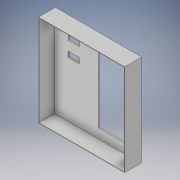
# Autodesk Inventor part: tetris body
Saved by Autodesk Inventor 2017 (Build 210142000, 142)
## iProperties
Created: 2019-08-23
Part Number: tetris body
Material: Generic
Document SubType Name: Modeling
Designer: EDMU0006
Density: 1 g/cm^3
Appearance: Default
Author: EDMU0006
Autodesk Inventor part; units mm, degrees
ref_plane "YZ Plane" through (0, 0, 0) normal (1, 0, 0) x (0, 1, 0)
ref_plane "XZ Plane" through (0, 0, 0) normal (0, 1, 0) x (-1, 0, 0)
ref_plane "XY Plane" through (0, 0, 0) normal (0, 0, 1) x (1, 0, 0)
sketch "Sketch1" plane through (0, 0, 0) normal (0, 0, 1) x (1, 0, 0)
  line L0 (-362.4815, -406.4) -> (399.5185, -406.4)
  line L1 (399.5185, -406.4) -> (399.5185, 406.4)
  line L2 (399.5185, 406.4) -> (-362.4815, 406.4)
  line L3 (-362.4815, 406.4) -> (-362.4815, -406.4)
  point P0 (0, 0)
  constraints: 8 end point, 2 perpendicular, 1 vertical
extrude "Extrusion1" add sketch "Sketch1" along normal blind 150.114
sketch "Sketch3" plane through (0, 0, 150.114) normal (0, 0, 1) x (1, 0, 0)
  line L0 (-356.7823, 401.8579) -> (395.0577, 401.8579)
  line L1 (395.0577, 401.8579) -> (395.0577, -400.7821)
  line L2 (395.0577, -400.7821) -> (-356.7823, -400.7821)
  line L3 (-356.7823, -400.7821) -> (-356.7823, 401.8579)
  point P0 (0, 0)
  dimension "d10" = 751.84
  dimension "d11" = 802.64
  constraints: 8 end point, 2 parallel, 1 horizontal, 1 perpendicular
  measures "d10" distance of L0.start L0.end
  measures "d11" distance of L0.end L1.end
extrude "Extrusion2" cut sketch "Sketch3" against normal blind 139.7
sketch "Sketch4" plane through (0, 0, 0) normal (0, 0, -1) x (-1, 0, 0)
  line L0 (-345.9489, 321.1782) -> (-25.9089, 321.1782)
  line L1 (-25.9089, 321.1782) -> (-25.9089, -318.9018)
  line L2 (-25.9089, -318.9018) -> (-345.9489, -318.9018)
  line L3 (-345.9489, -318.9018) -> (-345.9489, 321.1782)
  line L4 (140.3393, 137.685) -> (240.6693, 137.685)
  line L5 (240.6693, 137.685) -> (240.6693, 90.4401)
  line L6 (240.6693, 90.4401) -> (140.3393, 90.4401)
  line L7 (140.3393, 90.4401) -> (140.3393, 137.685)
  line L8 (139.7596, 266.0514) -> (240.0896, 266.0514)
  line L9 (240.0896, 266.0514) -> (240.0896, 218.8065)
  line L10 (240.0896, 218.8065) -> (139.7596, 218.8065)
  line L11 (139.7596, 218.8065) -> (139.7596, 266.0514)
  point P0 (0, 0)
  dimension "d17" = 100.33
  dimension "d18" = 47.2449
  dimension "d19" = 100.33
  dimension "d20" = 47.2449
  constraints: 24 end point, 6 parallel, 3 horizontal, 3 perpendicular
  measures "d17" distance of L5.end L6.end
  measures "d18" distance of L4.end L5.end
  measures "d19" distance of L10.start L10.end
  measures "d20" distance of L9.start L10.start
extrude "Extrusion3" cut sketch "Sketch4" against normal blind 279.4
body "Solid1"
